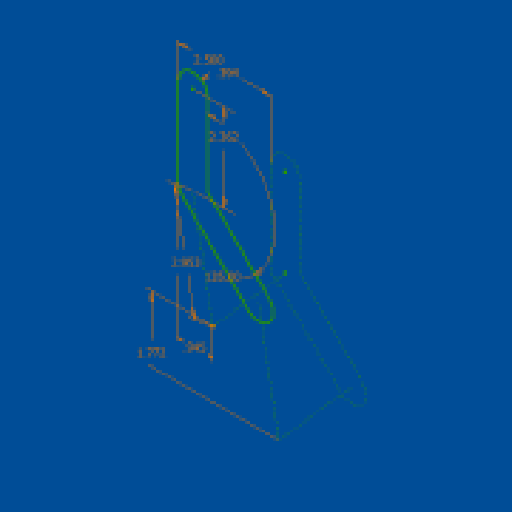
# Autodesk Inventor part: clawPanel
Saved by Autodesk Inventor 2023 (Build 270158030, 158C)
## iProperties
Created: 2023-03-03
Part Number: clawPanel
Material: Generic
Document SubType Name: Modeling
Designer: kumpu
Density: 1 g/cm^3
Appearance: Glossy - Black
Author: kumpu
Autodesk Inventor part; units mm, degrees
ref_plane "YZ Plane" through (0, 0, 0) normal (1, 0, 0) x (0, 1, 0)
ref_plane "XZ Plane" through (0, 0, 0) normal (0, 1, 0) x (-1, 0, 0)
ref_plane "XY Plane" through (0, 0, 0) normal (0, 0, 1) x (1, 0, 0)
sketch "Sketch1" plane through (0, 0, 0) normal (0, 0, 1) x (1, 0, 0)
  line L0 (-24, 73.6817) -> (-24, 133.6817)
  arc A0 (-4, 133.6817) -> (-24, 133.6817) centre (-14, 133.6817) ccw
  line L1 (-4, 133.6817) -> (-4, 77.8239)
  line L2 (-4, 77.8239) -> (38.0711, 35.7528)
  arc A1 (23.9289, 21.6107) -> (38.0711, 35.7528) centre (31, 28.6817) ccw
  line L3 (23.9289, 21.6107) -> (-21.0711, 66.6107)
  arc A2 (-24, 73.6817) -> (-21.0711, 66.6107) centre (-14, 73.6817) ccw
  line L4 (-14, 73.6817) -> (0, 0) construction
  line L5 (0, 0) -> (49.5, 56.3449) construction
  line L6 (39.5, 56.3449) -> (39.5, 116.3449) construction
  arc A3 (59.5, 116.3449) -> (39.5, 116.3449) centre (49.5, 116.3449) ccw construction
  line L7 (59.5, 116.3449) -> (59.5, 60.4871) construction
  line L8 (59.5, 60.4871) -> (101.5711, 18.416) construction
  arc A4 (87.4289, 4.2739) -> (101.5711, 18.416) centre (94.5, 11.3449) ccw construction
  line L9 (87.4289, 4.2739) -> (42.4289, 49.2739) construction
  arc A5 (39.5, 56.3449) -> (42.4289, 49.2739) centre (49.5, 56.3449) ccw construction
  line L10 (31, 28.6817) -> (45, -45) construction
  line L11 (45, -45) -> (94.5, 11.3449) construction
  circle A6 centre (-14, 133.6817) radius 2
  circle A7 centre (-14, 73.6817) radius 2
  circle A8 centre (31, 28.6817) radius 2
  line L12 (-14, 133.6817) -> (-14, 73.6817) construction
  circle A9 centre (-14, 103.6817) radius 2
  dimension "d0" = 10
  dimension "d1" = 24
  dimension "d2" = 63.5
  dimension "d3" = 60
  dimension "d4" = 75
  dimension "d5" = 135
  dimension "d7" = 45
  dimension "d8" = 4
  constraints: 28 end point, 12 point on circle, 12 tangent, 10 centre point, 8 equal radius, 5 coincident, 5 equal length, 5 parallel, 3 vertical, 1 midpoint
  measures "d0" radius of A0
  measures "d1" distance from line of point (0, 0) L0
  measures "d2" distance between parallel lines of L0 L6
  measures "d3" distance of L4.start A0.centre
  measures "d4" distance of L4.start L4.end
  measures "d5" angle of L1 L2
  measures "d7" horizontal distance of L4.end L10.end
  measures "d8" diameter of A6
extrude "Extrusion1" add sketch "Sketch1" along normal blind 3
body "Solid1"
